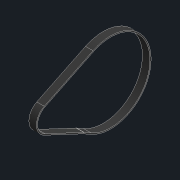
# Autodesk Inventor part: belt_2
Saved by Autodesk Inventor 2022 (Build 260153000, 153)
## iProperties
Created: 2021-07-18
Part Number: belt_2
Material: ゴム
Document SubType Name: Modeling
Designer: yuta0
Density: 0.93 g/cm^3
Appearance: ゴム - 黒
Mass: 8.55769 g
Surface Area: 248.449 cm^2
Volume: 9.20182 cm^3
購入先: ミスミ
在庫数: 0.0
Author: yuta0
Autodesk Inventor part; units mm, degrees
ref_plane "YZ Plane" through (0, 0, 0) normal (1, 0, 0) x (0, 1, 0)
ref_plane "XZ Plane" through (0, 0, 0) normal (0, 1, 0) x (-1, 0, 0)
ref_plane "XY Plane" through (0, 0, 0) normal (0, 0, 1) x (1, 0, 0)
sketch "スケッチ1" plane through (0, 0, 0) normal (1, 0, 0) x (0, 1, 0)
  arc A0 (15.7412, 7.6624) -> (-15.8575, 7.4187) centre (0, 0) ccw
  arc A1 (-45.5533, -53.8587) -> (47.2235, -57.0128) centre (0, -80) ccw
  arc A2 (-40.1767, -44.4895) -> (-39.8299, -43.8223) centre (-48, -40) ccw
  line L0 (-39.8299, -43.8223) -> (-15.8575, 7.4187)
  line L1 (47.2235, -57.0128) -> (15.7412, 7.6624)
  line L2 (-40.1767, -44.4895) -> (-45.5533, -53.8587)
  arc A3 (16.6583, 8.1088) -> (-16.7814, 7.8509) centre (0, 0) ccw
  line L3 (-16.7814, 7.8509) -> (-40.7538, -43.39)
  arc A4 (-41.0613, -43.9818) -> (-40.7538, -43.39) centre (-48, -40) ccw
  line L4 (-41.0613, -43.9818) -> (-46.438, -53.351)
  arc A5 (-46.438, -53.351) -> (48.1406, -56.5663) centre (0, -80) ccw
  line L5 (48.1406, -56.5663) -> (16.6583, 8.1088)
  arc A6 (15.3096, 7.4523) -> (-15.4227, 7.2153) centre (0, 0) ccw
  line L6 (-15.4227, 7.2153) -> (-39.3951, -44.0257)
  arc A7 (-39.7603, -44.7284) -> (-39.3951, -44.0257) centre (-48, -40) ccw
  line L7 (-39.7603, -44.7284) -> (-45.137, -54.0976)
  arc A8 (-45.137, -54.0976) -> (46.7919, -57.2228) centre (0, -80) ccw
  line L8 (46.7919, -57.2228) -> (15.3096, 7.4523)
  dimension "d0" = 35.0141
  dimension "d1" = 105.0423
  dimension "d2" = 80
  dimension "d25" = 8
  dimension "d26" = 40
  dimension "d30" = 48
  dimension "d31" = 1.5
  dimension "d32" = 0.48
  constraints: 18 end point, 18 point on circle, 9 centre point, 6 tangent, 1 coincident, 1 vertical alignment, 10 other
  measures "d0" diameter of A0
  measures "d1" diameter of A1
  measures "d2" distance of A0.centre A1.centre
  measures "d25" radius of A4
  measures "d26" vertical distance of point (0, 0) A2.centre
  measures "d30" horizontal distance of point (0, 0) A2.centre
  measures "d31" distance between parallel lines of L5 L8
  measures "d32" distance between parallel lines of L8 L1
extrude "押し出し1" add sketch "スケッチ1" along normal mid plane 10 contours L1 A1 L2 A2 L0 A0 | L5 A5 L4 A4 L3 A3
